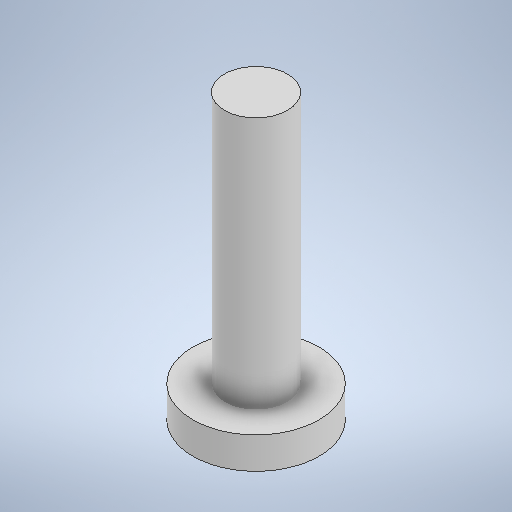
# Autodesk Inventor part: Taststift
Saved by Autodesk Inventor 2025 (Build 290162000, 162)
## iProperties
Created: 2026-07-12
Part Number: Taststift
Material: Generisch
Document SubType Name: Modeling
Designer: wavid
Mass: 0.991864 g
Surface Area: 10.1034 cm^2
Volume: 0.991864 cm^3
Density: 1 g/cm^3
Appearance: Vorgabe
Author: wavid
Autodesk Inventor part; units mm, degrees
ref_plane "YZ Plane" through (0, 0, 0) normal (1, 0, 0) x (0, 1, 0)
ref_plane "XZ Plane" through (0, 0, 0) normal (0, 1, 0) x (-1, 0, 0)
sketch "Skizze1" plane through (0, 0, 0) normal (0, 0, 1) x (1, 0, 0)
  circle A0 centre (0, 0) radius 3
  constraints: 1 centre point
extrude "Extrusion1" add sketch "Skizze1" along normal blind 27
sketch "Skizze2" plane through (0, 0, 0) normal (0, 0, 1) x (1, 0, 0)
  circle A0 centre (0, 0) radius 6
  constraints: 1 centre point
extrude "Extrusion2" add sketch "Skizze2" along normal blind 3 separate body
ref_plane "Arbeitsebene1" through (0, 0, 4) normal (0, 0, 1) x (1, 0, 0)
sketch "Skizze3" plane through (0, 0, 4) normal (0, 0, 1) x (1, 0, 0)
  circle A0 centre (0, 0) radius 2.1
  constraints: 1 centre point
extrude "Extrusion3" cut sketch "Skizze3" along normal mid plane 8 bodies 1
